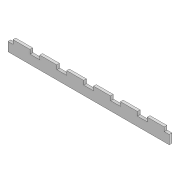
# Autodesk Inventor part: tray_side_support
Saved by Autodesk Inventor 2022 (Build 260153000, 153)
## iProperties
Created: 2022-05-19
Part Number: tray_side_support
Material: Generic
Document SubType Name: Modeling
Designer: Thomas
Density: 1 g/cm^3
Appearance: Default
Author: Thomas
Autodesk Inventor part; units mm, degrees
ref_plane "YZ Plane" through (0, 0, 0) normal (1, 0, 0) x (0, 1, 0)
ref_plane "XZ Plane" through (0, 0, 0) normal (0, 1, 0) x (-1, 0, 0)
ref_plane "XY Plane" through (0, 0, 0) normal (0, 0, 1) x (1, 0, 0)
sketch "Sketch1" plane through (0, 0, 0) normal (0, 0, 1) x (1, 0, 0)
  line L0 (0, 0) -> (180, 0)
  line L1 (180, 0) -> (180, -10)
  line L2 (180, -10) -> (0, -10)
  line L3 (0, -10) -> (0, 0)
  line L4 (5.5, 0) -> (24.5, 0)
  line L5 (24.5, 0) -> (24.5, 4.5)
  line L6 (24.5, 4.5) -> (5.5, 4.5)
  line L7 (5.5, 4.5) -> (5.5, 0)
  line L8 (54.5, 4.5) -> (35.5, 4.5)
  line L9 (54.5, 0) -> (54.5, 4.5)
  line L10 (35.5, 4.5) -> (35.5, 0)
  line L11 (84.5, 4.5) -> (65.5, 4.5)
  line L12 (84.5, 0) -> (84.5, 4.5)
  line L13 (65.5, 4.5) -> (65.5, 0)
  line L14 (114.5, 4.5) -> (95.5, 4.5)
  line L15 (114.5, 0) -> (114.5, 4.5)
  line L16 (95.5, 4.5) -> (95.5, 0)
  line L17 (144.5, 4.5) -> (125.5, 4.5)
  line L18 (144.5, 0) -> (144.5, 4.5)
  line L19 (125.5, 4.5) -> (125.5, 0)
  line L20 (174.5, 4.5) -> (155.5, 4.5)
  line L21 (174.5, 0) -> (174.5, 4.5)
  line L22 (155.5, 4.5) -> (155.5, 0)
  dimension "d0" = 180
  dimension "d1" = 10
  dimension "d2" = 19
  dimension "d3" = 4.5
  dimension "d4" = 5.5
  dimension "d7" = 30
  constraints: 46 end point, 4 parallel, 3 horizontal, 2 perpendicular, 1 point on line, 35 other
  measures "d0" distance of L1.end L2.end
  measures "d1" distance of L0.end L1.end
  measures "d2" distance of L6.end L5.end
  measures "d3" distance of L5.end L4.end
  measures "d4" distance between parallel lines of L7 L3
  measures "d7" distance of L5.end L8.start
extrude "Extrusion1" add sketch "Sketch1" along normal blind 3
body "Solid1"
